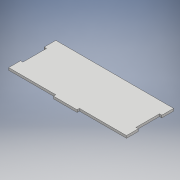
# Autodesk Inventor part: bawah
Saved by Autodesk Inventor 2017 (Build 210142000, 142)
## iProperties
Created: 2017-01-06
Part Number: bawah
Material: Generic
Document SubType Name: Modeling
Designer: Ghesa Bhakti
Density: 1 g/cm^3
Appearance: Default
Author: Ghesa Bhakti
Autodesk Inventor part; units mm, degrees
ref_plane "YZ Plane" through (0, 0, 0) normal (1, 0, 0) x (0, 1, 0)
ref_plane "XZ Plane" through (0, 0, 0) normal (0, 1, 0) x (-1, 0, 0)
ref_plane "XY Plane" through (0, 0, 0) normal (0, 0, 1) x (1, 0, 0)
sketch "Sketch1" plane through (0, 0, 0) normal (0, 0, 1) x (1, 0, 0)
  line L0 (90, 0) -> (90, -3)
  line L1 (90, -3) -> (60, -3)
  line L2 (60, -3) -> (60, 0)
  line L3 (0, 0) -> (60, 0)
  line L4 (90, 0) -> (150, 0)
  line L5 (0, 45) -> (3, 45)
  line L6 (3, 45) -> (3, 15)
  line L7 (3, 15) -> (0, 15)
  line L8 (0, 60) -> (0, 45)
  line L9 (0, 15) -> (0, 0)
  line L10 (150, 60) -> (0, 60)
  line L11 (150, 15) -> (147, 15)
  line L12 (147, 15) -> (147, 45)
  line L13 (147, 45) -> (150, 45)
  line L14 (150, 0) -> (150, 15)
  line L15 (150, 45) -> (150, 60)
  dimension "d1" = 150
  dimension "d2" = 60
  dimension "d6" = 3
  dimension "d7" = 15
  dimension "d8" = 3
  dimension "d10" = 30
  dimension "d11" = 30
  dimension "d12" = 3
  dimension "d13" = 3
  dimension "d14" = 15
  constraints: 32 end point, 5 horizontal, 3 parallel, 2 perpendicular, 2 vertical
  measures "d1" distance of L9.end L4.end
  measures "d2" distance of L8.start L9.end
  measures "d6" distance of L0.start L0.end
  measures "d7" distance of L8.start L8.end
  measures "d8" distance of L6.end L7.end
  measures "d10" distance of L0.end L2.start
  measures "d11" distance of L11.end L12.end
  measures "d12" distance of L11.start L11.end
  measures "d13" distance of L12.end L13.end
  measures "d14" distance of L4.end L11.start
extrude "Extrusion1" add sketch "Sketch1" along normal blind 3
body "Solid1"
